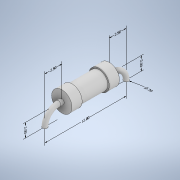
# Autodesk Inventor part: Деталь3-01
Saved by Autodesk Inventor 2021 (Build 250183000, 183)
## iProperties
Created: 2022-10-18
Part Number: Деталь3-01
Material: Типовые
Document SubType Name: Modeling
Designer: 22-91-12
Density: 1 g/cm^3
Appearance: По умолчанию
Author: 22-91-12
Autodesk Inventor part; units mm, degrees
ref_plane "YZ Plane" through (0, 0, 0) normal (1, 0, 0) x (0, 1, 0)
ref_plane "XZ Plane" through (0, 0, 0) normal (0, 1, 0) x (-1, 0, 0)
ref_plane "XY Plane" through (0, 0, 0) normal (0, 0, 1) x (1, 0, 0)
sketch "Эскиз1" plane through (0, 0, 0) normal (0, 1, 0) x (-1, 0, 0)
  line L0 (4.0742, 9.2484) -> (4.0742, 7.7484)
  line L1 (4.0742, 7.7484) -> (3.8742, 7.7484)
  line L2 (3.8742, 7.7484) -> (3.8742, 3.7484)
  line L3 (3.8742, 3.7484) -> (4.0742, 3.7484)
  line L4 (4.0742, 3.7484) -> (4.0742, 2.2484)
  line L5 (4.0742, 2.2484) -> (2.5742, 2.2484)
  line L6 (2.5742, 2.2484) -> (2.5742, 9.2484)
  line L7 (2.5742, 9.2484) -> (4.0742, 9.2484)
  point P0 (0, 0)
  dimension "d0" = 1.5
  dimension "d1" = 0.2
  dimension "d2" = 4
  dimension "d3" = 0.2
  dimension "d4" = 1.5
  dimension "d5" = 1.5
  dimension "d6" = 7
  constraints: 16 end point, 3 perpendicular, 2 point on line, 2 vertical
  measures "d0" distance of L0.start L0.end
  measures "d1" distance of L0.end L1.end
  measures "d2" distance of L1.end L2.end
  measures "d3" distance of L2.end L3.end
  measures "d4" distance of L3.end L4.end
  measures "d5" distance of L4.end L5.end
  measures "d6" distance of L5.end L6.end
revolve "Вращение1" add sketch "Эскиз1" angle 360 about axis through (-2.5742, 0, 2.2484) along (0, 0, 1)
sketch "Эскиз2" plane through (-2.5742, 0, 9.2484) normal (0, 0, 1) x (1, 0, 0)
  circle A0 centre (0, 0) radius 1.3 projected
  circle A1 centre (0, 0) radius 0.35
  circle A2 centre (-6.8053, 0) radius 0.3139
  point P0 (2.5742, 0)
  dimension "d8" = 0.7
  constraints: 2 centre point, 1 coincident
  measures "d8" diameter of A1
sketch "Эскиз3" plane through (-2.5742, 0, 2.2484) normal (0, 0, -1) x (-1, 0, 0)
  circle A0 centre (0, 0) radius 0.35
  point P0 (-2.5742, 0)
  dimension "d9" = 0.7
  constraints: 1 centre point
  measures "d9" diameter of A0
sketch3d "3D эскиз1"
  line L0 (-2.5742, 0, 2.2484) -> (-2.5742, 0, 1.7484)
  arc A0 (-2.5742, 0, 1.7484) -> (-2.5742, -2, -0.2516) centre (-2.5742, -2, 1.7484) ccw
  dimension "d10" = 2.5
  dimension "d11" = 2
  dimension "d16" = 2
sweep "Сдвиг2" add profiles "Эскиз3" path "3D эскиз1"
sketch3d "3D эскиз2"
  line L0 (-2.5742, 0, 9.2484) -> (-2.5742, 0, 9.7484)
  arc A0 (-2.5742, 0, 9.7484) -> (-2.5742, -2, 11.7484) centre (-2.5742, -2, 9.7484) ccw
  dimension "d12" = 2.5
  dimension "d13" = 2
  dimension "d19" = 2
sweep "Сдвиг3" add profiles "Эскиз2" path "3D эскиз2" contours A1
equation "\"D22\" = d10 + d6 + d12"
